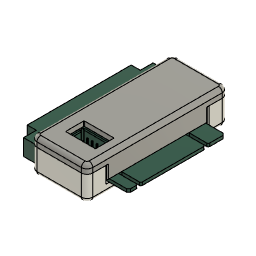
C64_Wifi_PET_adapter v4 (Autodesk Fusion 360 design; units mm, degrees)
Autodesk Fusion 360 part; units mm, degrees
sketch "pcb" plane through (0, 0, 0) normal (0, 0, 1) x (1, 0, 0) in component "PCB"
  arc A0 (28, 1.5) -> (27, 0.5) centre (28, 0.5) ccw
  line L0 (27, 0) -> (27, 0.5)
  line L1 (0, 54) -> (27, 54)
  line L2 (0, 54) -> (0, 0)
  line L3 (28, 1.5) -> (39, 1.5)
  line L4 (39.2, 42.04) -> (30, 42.04)
  line L5 (40, 51.5) -> (40, 44.44)
  line L6 (39, 1.5) -> (40, 2.5)
  line L7 (40, 4.12) -> (40, 5.6)
  arc A1 (30, 8) -> (29.2, 7.2) centre (30, 7.2) ccw
  arc A2 (29.2, 42.84) -> (30, 42.04) centre (30, 42.84) ccw
  arc A3 (30, 43.64) -> (29.2, 42.84) centre (30, 42.84) ccw
  line L8 (40, 4.12) -> (40, 2.5)
  arc A4 (40, 41.24) -> (39.2, 42.04) centre (39.2, 41.24) ccw
  arc A5 (29.2, 7.2) -> (30, 6.4) centre (30, 7.2) ccw
  line L9 (30, 8) -> (39.2, 8)
  line L10 (30, 43.64) -> (39.2, 43.64)
  line L11 (28, 52.5) -> (39, 52.5)
  arc A6 (39.2, 8) -> (40, 8.8) centre (39.2, 8.8) ccw
  arc A7 (27, 53.5) -> (28, 52.5) centre (28, 53.5) ccw
  arc A8 (39.2, 43.64) -> (40, 44.44) centre (39.2, 44.44) ccw
  line L12 (39, 52.5) -> (40, 51.5)
  line L13 (40, 8.8) -> (40, 41.24)
  line L14 (27, 54) -> (27, 53.5)
  line L15 (39.2, 6.4) -> (30, 6.4)
  arc A9 (40, 5.6) -> (39.2, 6.4) centre (39.2, 5.6) ccw
  line L16 (0, 0) -> (27, 0)
  line L17 (0.1, 41.86) -> (4, 41.86)
  line L18 (18.794, 6.016) -> (18.794, 6.524)
  line L19 (0.1, 35.9) -> (4, 35.9)
  line L20 (0.1, 43.82) -> (4, 43.82)
  line L21 (3, 49.28) -> (2, 49.28)
  arc A10 (4, 43.82) -> (4, 45.82) centre (4, 44.82) ccw
  arc A11 (4, 35.9) -> (4, 37.9) centre (4, 36.9) ccw
  line L22 (16.254, 3.476) -> (16.254, 3.984)
  line L23 (3, 41.36) -> (2, 41.36)
  line L24 (16.254, 3.984) -> (15.746, 3.984)
  line L25 (0.1, 45.82) -> (4, 45.82)
  line L26 (18.794, 3.476) -> (18.794, 3.984)
  arc A12 (3, 36.4) -> (3, 37.4) centre (3, 36.9) ccw
  line L27 (13.206, 6.016) -> (13.714, 6.016)
  line L28 (13.714, 3.476) -> (13.714, 3.984)
  arc A13 (3, 44.32) -> (3, 45.32) centre (3, 44.82) ccw
  arc A14 (2, 45.32) -> (2, 44.32) centre (2, 44.82) ccw
  line L29 (18.794, 3.984) -> (18.286, 3.984)
  line L30 (0.1, 37.9) -> (4, 37.9)
  line L31 (18.794, 6.524) -> (18.286, 6.524)
  line L32 (15.746, 6.524) -> (15.746, 6.016)
  line L33 (13.714, 6.524) -> (13.206, 6.524)
  line L34 (0.1, 49.78) -> (4, 49.78)
  line L35 (0.1, 39.86) -> (4, 39.86)
  line L36 (13.714, 3.984) -> (13.206, 3.984)
  line L37 (18.286, 6.524) -> (18.286, 6.016)
  line L38 (18.286, 3.984) -> (18.286, 3.476)
  line L39 (3, 37.4) -> (2, 37.4)
  line L40 (15.746, 6.016) -> (16.254, 6.016)
  line L41 (13.714, 6.016) -> (13.714, 6.524)
  line L42 (3, 48.28) -> (2, 48.28)
  arc A15 (2, 41.36) -> (2, 40.36) centre (2, 40.86) ccw
  arc A16 (4, 39.86) -> (4, 41.86) centre (4, 40.86) ccw
  arc A17 (3, 48.28) -> (3, 49.28) centre (3, 48.78) ccw
  arc A18 (3, 40.36) -> (3, 41.36) centre (3, 40.86) ccw
  line L43 (13.206, 6.524) -> (13.206, 6.016)
  arc A19 (2, 37.4) -> (2, 36.4) centre (2, 36.9) ccw
  line L44 (16.254, 6.524) -> (15.746, 6.524)
  line L45 (0.1, 47.78) -> (4, 47.78)
  arc A20 (2, 49.28) -> (2, 48.28) centre (2, 48.78) ccw
  line L46 (3, 44.32) -> (2, 44.32)
  line L47 (3, 36.4) -> (2, 36.4)
  line L48 (13.206, 3.476) -> (13.714, 3.476)
  line L49 (3, 40.36) -> (2, 40.36)
  line L50 (13.206, 3.984) -> (13.206, 3.476)
  arc A21 (4, 47.78) -> (4, 49.78) centre (4, 48.78) ccw
  line L51 (15.746, 3.476) -> (16.254, 3.476)
  line L52 (15.746, 3.984) -> (15.746, 3.476)
  line L53 (18.286, 6.016) -> (18.794, 6.016)
  line L54 (16.254, 6.016) -> (16.254, 6.524)
  line L55 (18.286, 3.476) -> (18.794, 3.476)
  line L56 (3, 45.32) -> (2, 45.32)
  line L57 (3, 32.44) -> (2, 32.44)
  arc A22 (2, 17.6) -> (2, 16.6) centre (2, 17.1) ccw
  line L58 (3, 29.48) -> (2, 29.48)
  arc A23 (3, 8.68) -> (3, 9.68) centre (3, 9.18) ccw
  line L59 (3, 25.52) -> (2, 25.52)
  line L60 (0.1, 14.14) -> (4, 14.14)
  line L61 (0.1, 24.02) -> (4, 24.02)
  arc A24 (2, 33.44) -> (2, 32.44) centre (2, 32.94) ccw
  line L62 (3, 12.64) -> (2, 12.64)
  line L63 (0.1, 6.22) -> (4, 6.22)
  arc A25 (4, 16.1) -> (4, 18.1) centre (4, 17.1) ccw
  line L64 (0.1, 20.06) -> (4, 20.06)
  arc A26 (2, 29.48) -> (2, 28.48) centre (2, 28.98) ccw
  line L65 (0.1, 29.98) -> (4, 29.98)
  arc A27 (3, 20.56) -> (3, 21.56) centre (3, 21.06) ccw
  line L66 (0.1, 10.18) -> (4, 10.18)
  arc A28 (4, 24.02) -> (4, 26.02) centre (4, 25.02) ccw
  arc A29 (3, 24.52) -> (3, 25.52) centre (3, 25.02) ccw
  arc A30 (4, 27.98) -> (4, 29.98) centre (4, 28.98) ccw
  line L67 (3, 9.68) -> (2, 9.68)
  arc A31 (2, 13.64) -> (2, 12.64) centre (2, 13.14) ccw
  line L68 (3, 20.56) -> (2, 20.56)
  line L69 (0.1, 33.94) -> (4, 33.94)
  line L70 (3, 5.72) -> (2, 5.72)
  line L71 (3, 16.6) -> (2, 16.6)
  arc A32 (3, 12.64) -> (3, 13.64) centre (3, 13.14) ccw
  arc A33 (2, 5.72) -> (2, 4.72) centre (2, 5.22) ccw
  line L72 (0.1, 16.1) -> (4, 16.1)
  arc A34 (2, 21.56) -> (2, 20.56) centre (2, 21.06) ccw
  line L73 (3, 8.68) -> (2, 8.68)
  arc A35 (4, 20.06) -> (4, 22.06) centre (4, 21.06) ccw
  line L74 (0.1, 12.14) -> (4, 12.14)
  line L75 (3, 4.72) -> (2, 4.72)
  line L76 (0.1, 8.18) -> (4, 8.18)
  arc A36 (2, 25.52) -> (2, 24.52) centre (2, 25.02) ccw
  arc A37 (4, 12.14) -> (4, 14.14) centre (4, 13.14) ccw
  arc A38 (2, 9.68) -> (2, 8.68) centre (2, 9.18) ccw
  line L77 (0.1, 31.94) -> (4, 31.94)
  arc A39 (4, 31.94) -> (4, 33.94) centre (4, 32.94) ccw
  arc A40 (4, 8.18) -> (4, 10.18) centre (4, 9.18) ccw
  arc A41 (4, 4.22) -> (4, 6.22) centre (4, 5.22) ccw
  line L78 (3, 21.56) -> (2, 21.56)
  line L79 (0.1, 18.1) -> (4, 18.1)
  arc A42 (3, 28.48) -> (3, 29.48) centre (3, 28.98) ccw
  arc A43 (3, 4.72) -> (3, 5.72) centre (3, 5.22) ccw
  arc A44 (3, 16.6) -> (3, 17.6) centre (3, 17.1) ccw
  line L80 (0.1, 4.22) -> (4, 4.22)
  line L81 (3, 13.64) -> (2, 13.64)
  line L82 (0.1, 27.98) -> (4, 27.98)
  line L83 (3, 24.52) -> (2, 24.52)
  line L84 (3, 28.48) -> (2, 28.48)
  arc A45 (3, 32.44) -> (3, 33.44) centre (3, 32.94) ccw
  line L85 (3, 17.6) -> (2, 17.6)
  line L86 (0.1, 26.02) -> (4, 26.02)
  line L87 (3, 33.44) -> (2, 33.44)
  line L88 (0.1, 22.06) -> (4, 22.06)
  line L89 (14.73, 1.6662) -> (14.73, 1.19)
  line L90 (23.62, 6.7463) -> (23.62, 0.3962)
  arc A46 (22.35, 9.6038) -> (21.08, 9.6038) centre (21.715, 9.6038) ccw
  line L91 (14.73, 1.6662) -> (9.65, 1.6662)
  line L92 (9.1737, 6.7463) -> (9.1737, 1.19)
  line L93 (8.38, 8.175) -> (8.38, 9.6038)
  line L94 (14.73, 1.19) -> (14.73, 0.3962)
  line L95 (22.35, 1.6662) -> (22.8263, 1.19)
  line L96 (22.35, 8.175) -> (22.35, 6.7463)
  line L97 (9.65, 8.175) -> (9.1737, 8.175)
  line L98 (22.8263, 8.175) -> (22.8263, 8.81)
  line L99 (9.1737, 1.19) -> (9.65, 1.6662)
  line L100 (9.1737, 8.81) -> (9.65, 8.3338)
  line L101 (22.35, 8.175) -> (22.8263, 8.175)
  line L102 (8.38, 0.3962) -> (8.38, 6.7463)
  line L103 (14.73, 1.19) -> (9.1737, 1.19)
  line L104 (23.62, 9.6038) -> (23.62, 8.175)
  arc A47 (10.92, 9.6038) -> (9.65, 9.6038) centre (10.285, 9.6038) ccw
  line L105 (22.8263, 8.175) -> (23.62, 8.175)
  line L106 (22.35, 6.7463) -> (22.8263, 6.7463)
  line L107 (9.65, 1.6662) -> (9.65, 6.7463)
  line L108 (9.1737, 8.81) -> (9.1737, 8.175)
  arc A48 (16.4763, 9.6038) -> (15.3651, 9.6038) centre (15.9207, 9.6038) ccw
  line L109 (22.35, 1.6662) -> (17.27, 1.6662)
  line L110 (9.65, 8.3338) -> (22.35, 8.3338)
  line L111 (22.8263, 6.7463) -> (22.8263, 1.19)
  line L112 (17.27, 1.19) -> (22.8263, 1.19)
  line L113 (22.35, 6.7463) -> (22.35, 1.6662)
  line L114 (9.1737, 8.175) -> (8.38, 8.175)
  line L115 (0.1, 20.06) -> (-1, 20.06)
  line L116 (0.1, 49.78) -> (-1, 49.78)
  line L117 (-1, 53.8) -> (0, 53.8)
  line L118 (0, 27.25) -> (-1, 27.25)
  line L119 (-1, 14.87) -> (0, 14.87)
  line L120 (0.1, 35.9) -> (-1, 35.9)
  line L121 (0, 50.51) -> (0, 51.01)
  line L122 (0, 42.59) -> (0, 43.09)
  line L123 (0.1, 41.86) -> (-1, 41.86)
  line L124 (0.1, 47.78) -> (-1, 47.78)
  line L125 (0, 61.25) -> (-6.8, 61.25)
  line L126 (-1, 18.83) -> (0, 18.83)
  line L127 (0.1, 43.82) -> (-1, 43.82)
  line L128 (0, 31.21) -> (-1, 31.21)
  line L129 (0, -7.25) -> (-6.8, -7.25)
  line L130 (0, 23.29) -> (-1, 23.29)
  line L131 (0.1, 14.14) -> (-1, 14.14)
  line L132 (0.1, 29.98) -> (-1, 29.98)
  line L133 (-1, 42.59) -> (0, 42.59)
  line L134 (0, 59.7) -> (0, 61.25)
  line L135 (0, 0.2) -> (-1, 0.2)
  line L136 (0.1, 22.06) -> (-1, 22.06)
  line L137 (0.1, 39.86) -> (-1, 39.86)
  line L138 (0, 15.37) -> (-1, 15.37)
  line L139 (0, 58) -> (-2.8667, 58)
  line L140 (-1.6, -2.3) -> (0, -2.3)
  line L141 (0, 51.01) -> (-1, 51.01)
  line L142 (-6.8, 56.3) -> (-6.8, 59.7)
  line L143 (0, -2.3) -> (0, 0.2)
  line L144 (0.1, 45.82) -> (-1, 45.82)
  line L145 (0, 56.3) -> (0, 58)
  line L146 (0, -5.7) -> (0, -4)
  line L147 (-11.6, 54.5) -> (-6.8, 54.5)
  line L148 (0, 19.33) -> (-1, 19.33)
  line L149 (-1, 30.71) -> (0, 30.71)
  line L150 (-1, 50.51) -> (0, 50.51)
  line L151 (0, 43.09) -> (-1, 43.09)
  line L152 (0, -7.25) -> (0, -5.7)
  line L153 (0, 46.55) -> (0, 47.05)
  line L154 (-1, 0.2) -> (-1, 53.8)
  line L155 (-1, 38.63) -> (0, 38.63)
  line L156 (0, 39.13) -> (-1, 39.13)
  line L157 (0.1, 37.9) -> (-1, 37.9)
  line L158 (-1, 46.55) -> (0, 46.55)
  line L159 (0, 53.8) -> (0, 56.3)
  line L160 (-11.6, -4) -> (-8.7333, -4)
  line L161 (0.1, 18.1) -> (-1, 18.1)
  line L162 (0.1, 24.02) -> (-1, 24.02)
  line L163 (-11.6, -0.5) -> (-11.6, 54.5)
  line L164 (0, 38.63) -> (0, 39.13)
  line L165 (0, 58) -> (0, 59.7)
  line L166 (0, 47.05) -> (-1, 47.05)
  line L167 (-3.548, 58) -> (-3.6853, 58)
  line L168 (-6.8, 54.5) -> (-6.8, 56.3)
  line L169 (0.1, 26.02) -> (-1, 26.02)
  line L170 (0, -4) -> (0, -2.3)
  line L171 (-1, 22.79) -> (0, 22.79)
  line L172 (0.1, 27.98) -> (-1, 27.98)
  line L173 (0, 26.75) -> (0, 27.25)
  line L174 (-8.7333, 58) -> (-11.6, 58)
  line L175 (-6.8, -2.3) -> (-5.2, -2.3)
  line L176 (-4.2, -5.7) -> (-2.6, -5.7)
  line L177 (-3.6853, -4) -> (-3.548, -4)
  line L178 (-6.8, 56.3) -> (-5.2, 56.3)
  line L179 (22.35, 8.3338) -> (22.35, 8.175)
  line L180 (9.65, 8.175) -> (9.65, 8.3338)
  line L181 (22.35, 8.3338) -> (22.8263, 8.81)
  line L182 (-6.8, -7.25) -> (-6.8, -5.7)
  line L183 (17.27, 1.19) -> (17.27, 0.3962)
  line L184 (9.1737, 8.81) -> (22.8263, 8.81)
  line L185 (8.38, 6.7463) -> (8.38, 8.175)
  line L186 (-4.2, 56.3) -> (-2.6, 56.3)
  line L187 (9.65, 6.7463) -> (9.1737, 6.7463)
  line L188 (-6.8, -0.5) -> (-11.6, -0.5)
  line L189 (-6.8, -2.3) -> (-6.8, -0.5)
  line L190 (23.62, 0.3962) -> (17.27, 0.3962)
  line L191 (9.1737, 6.7463) -> (8.38, 6.7463)
  line L192 (-1.6, 59.7) -> (0, 59.7)
  line L193 (-4.2, 59.7) -> (-2.6, 59.7)
  line L194 (17.27, 1.6662) -> (14.73, 1.6662)
  line L195 (-8.052, -4) -> (-7.9147, -4)
  line L196 (8.38, 9.6038) -> (23.62, 9.6038)
  line L197 (14.73, 0.3962) -> (8.38, 0.3962)
  line L198 (-2.8667, -4) -> (0, -4)
  line L199 (-6.8, 59.7) -> (-5.2, 59.7)
  line L200 (-6.8, -5.7) -> (-5.2, -5.7)
  line L201 (9.65, 6.7463) -> (9.65, 8.175)
  line L202 (-4.2, -2.3) -> (-2.6, -2.3)
  line L203 (22.8263, 6.7463) -> (23.62, 6.7463)
  line L204 (17.27, 1.6662) -> (17.27, 1.19)
  line L205 (23.62, 8.175) -> (23.62, 6.7463)
  line L206 (17.27, 0.3962) -> (14.73, 0.3962)
  line L207 (-1.6, -5.7) -> (0, -5.7)
  line L208 (-6.8, 59.7) -> (-6.8, 61.25)
  line L209 (-7.2333, -4) -> (-4.3667, -4)
  line L210 (-7.9147, 58) -> (-8.052, 58)
  line L211 (-4.3667, 58) -> (-7.2333, 58)
  line L212 (-1.6, 56.3) -> (0, 56.3)
  line L213 (-6.8, -5.7) -> (-6.8, -2.3)
  line L214 (0.1, 8.18) -> (-1, 8.18)
  line L215 (0, 11.41) -> (-1, 11.41)
  line L216 (0.1, 12.14) -> (-1, 12.14)
  line L217 (0, 6.95) -> (0, 7.45)
  line L218 (0.1, 10.18) -> (-1, 10.18)
  line L219 (0.1, 4.22) -> (-1, 4.22)
  line L220 (0, 7.45) -> (-1, 7.45)
  line L221 (0.1, 6.22) -> (-1, 6.22)
  line L222 (-1, 2.99) -> (0, 2.99)
  line L223 (0, 2.99) -> (0, 3.49)
  line L224 (0.1, 16.1) -> (-1, 16.1)
  line L225 (-1, 10.91) -> (0, 10.91)
  line L226 (-1, 26.75) -> (0, 26.75)
  line L227 (-1, 34.67) -> (0, 34.67)
  line L228 (-1, 6.95) -> (0, 6.95)
  line L229 (0, 34.67) -> (0, 35.17)
  line L230 (0, 35.17) -> (-1, 35.17)
  line L231 (0, 3.49) -> (-1, 3.49)
  line L232 (0, 18.83) -> (0, 19.33)
  line L233 (0.1, 31.94) -> (-1, 31.94)
  line L234 (0, 22.79) -> (0, 23.29)
  line L235 (0.1, 33.94) -> (-1, 33.94)
  line L236 (0, 30.71) -> (0, 31.21)
  line L237 (0, 14.87) -> (0, 15.37)
  line L238 (0, 10.91) -> (0, 11.41)
  arc A49 (3, 48.28) -> (3, 49.28) centre (3, 48.78) ccw
  line L239 (3, 37.4) -> (2, 37.4)
  arc A50 (2, 41.36) -> (2, 40.36) centre (2, 40.86) ccw
  line L240 (0.1, 33.94) -> (4, 33.94)
  line L241 (3, 32.44) -> (2, 32.44)
  arc A51 (4, 39.86) -> (4, 41.86) centre (4, 40.86) ccw
  arc A52 (3, 32.44) -> (3, 33.44) centre (3, 32.94) ccw
  arc A53 (4, 31.94) -> (4, 33.94) centre (4, 32.94) ccw
  line L242 (3, 33.44) -> (2, 33.44)
  arc A54 (2, 45.32) -> (2, 44.32) centre (2, 44.82) ccw
  line L243 (0.1, 31.94) -> (4, 31.94)
  arc A55 (2, 49.28) -> (2, 48.28) centre (2, 48.78) ccw
  line L244 (0.1, 29.98) -> (4, 29.98)
  line L245 (0.1, 35.9) -> (4, 35.9)
  line L246 (3, 41.36) -> (2, 41.36)
  arc A56 (4, 35.9) -> (4, 37.9) centre (4, 36.9) ccw
  line L247 (0.1, 41.86) -> (4, 41.86)
  arc A57 (4, 43.82) -> (4, 45.82) centre (4, 44.82) ccw
  line L248 (0.1, 37.9) -> (4, 37.9)
  arc A58 (3, 44.32) -> (3, 45.32) centre (3, 44.82) ccw
  line L249 (0.1, 4.22) -> (4, 4.22)
  arc A59 (2, 21.56) -> (2, 20.56) centre (2, 21.06) ccw
  arc A60 (3, 24.52) -> (3, 25.52) centre (3, 25.02) ccw
  arc A61 (2, 33.44) -> (2, 32.44) centre (2, 32.94) ccw
  line L250 (3, 49.28) -> (2, 49.28)
  line L251 (3, 36.4) -> (2, 36.4)
  line L252 (3, 40.36) -> (2, 40.36)
  arc A62 (2, 37.4) -> (2, 36.4) centre (2, 36.9) ccw
  line L253 (0.1, 43.82) -> (4, 43.82)
  line L254 (0.1, 49.78) -> (4, 49.78)
  line L255 (3, 45.32) -> (2, 45.32)
  line L256 (0.1, 45.82) -> (4, 45.82)
  arc A63 (4, 47.78) -> (4, 49.78) centre (4, 48.78) ccw
  line L257 (0.1, 47.78) -> (4, 47.78)
  arc A64 (3, 28.48) -> (3, 29.48) centre (3, 28.98) ccw
  arc A65 (3, 40.36) -> (3, 41.36) centre (3, 40.86) ccw
  line L258 (0.1, 22.06) -> (4, 22.06)
  line L259 (0.1, 10.18) -> (4, 10.18)
  line L260 (3, 44.32) -> (2, 44.32)
  line L261 (0.1, 8.18) -> (4, 8.18)
  arc A66 (2, 13.64) -> (2, 12.64) centre (2, 13.14) ccw
  line L262 (3, 17.6) -> (2, 17.6)
  line L263 (3, 12.64) -> (2, 12.64)
  arc A67 (3, 36.4) -> (3, 37.4) centre (3, 36.9) ccw
  arc A68 (4, 8.18) -> (4, 10.18) centre (4, 9.18) ccw
  line L264 (3, 48.28) -> (2, 48.28)
  line L265 (0.1, 39.86) -> (4, 39.86)
  arc A69 (2, 29.48) -> (2, 28.48) centre (2, 28.98) ccw
  arc A70 (2, 9.68) -> (2, 8.68) centre (2, 9.18) ccw
  arc A71 (3, 4.72) -> (3, 5.72) centre (3, 5.22) ccw
  line L266 (0.1, 14.14) -> (4, 14.14)
  line L267 (3, 9.68) -> (2, 9.68)
  line L268 (0.1, 27.98) -> (4, 27.98)
  line L269 (3, 21.56) -> (2, 21.56)
  line L270 (0.1, 24.02) -> (4, 24.02)
  arc A72 (4, 16.1) -> (4, 18.1) centre (4, 17.1) ccw
  line L271 (0.1, 16.1) -> (4, 16.1)
  line L272 (0.1, 12.14) -> (4, 12.14)
  arc A73 (3, 12.64) -> (3, 13.64) centre (3, 13.14) ccw
  line L273 (3, 13.64) -> (2, 13.64)
  line L274 (3, 29.48) -> (2, 29.48)
  arc A74 (3, 8.68) -> (3, 9.68) centre (3, 9.18) ccw
  line L275 (3, 16.6) -> (2, 16.6)
  line L276 (0.1, 26.02) -> (4, 26.02)
  arc A75 (4, 20.06) -> (4, 22.06) centre (4, 21.06) ccw
  arc A76 (3, 16.6) -> (3, 17.6) centre (3, 17.1) ccw
  line L277 (3, 8.68) -> (2, 8.68)
  arc A77 (2, 25.52) -> (2, 24.52) centre (2, 25.02) ccw
  line L278 (3, 5.72) -> (2, 5.72)
  line L279 (0.1, 18.1) -> (4, 18.1)
  arc A78 (3, 20.56) -> (3, 21.56) centre (3, 21.06) ccw
  line L280 (3, 25.52) -> (2, 25.52)
  arc A79 (4, 27.98) -> (4, 29.98) centre (4, 28.98) ccw
  line L281 (0.1, 20.06) -> (4, 20.06)
  arc A80 (2, 17.6) -> (2, 16.6) centre (2, 17.1) ccw
  line L282 (0.1, 6.22) -> (4, 6.22)
  arc A81 (2, 5.72) -> (2, 4.72) centre (2, 5.22) ccw
  arc A82 (4, 12.14) -> (4, 14.14) centre (4, 13.14) ccw
  line L283 (3, 28.48) -> (2, 28.48)
  line L284 (3, 20.56) -> (2, 20.56)
  line L285 (3, 4.72) -> (2, 4.72)
  line L286 (3, 24.52) -> (2, 24.52)
  arc A83 (4, 4.22) -> (4, 6.22) centre (4, 5.22) ccw
  arc A84 (4, 24.02) -> (4, 26.02) centre (4, 25.02) ccw
  point P0 (16, 5)
  point P1 (0.4763, 51.9113)
  point P2 (0, 27)
  point P3 (40, 27)
extrude "Extrude1" add sketch "pcb" against normal blind 1.6 contours A0 L0 L1 L2 L3 L4 L5 L6 L7 A1 A2 A3 L8 A4 A5 L9 L10 L11 A6 A7 A8 L12 L13 L14 L15 A9 L16 L17 L19 L20 A10 A11 L25 L30 L34 L35 A16 L45 A21 L60 L61 L63 A25 L64 L65 L66 A28 A30 L69 L72 A35 L74 L76 A37 L77 A39 A40 A41 L79 L80 L82 L86 L88 L115 L116 L120 L121 L122 L123 L124 L127 L131 L132 L136 L137 L143 L144 L153 L157 L159 L161 L162 L164 L169 L172 L173 L214 L216 L217 L218 L219 L221 L223 L224 L229 L232 L233 L234 L235 L236 L237 L238 L240 A51 A53 L243 L244 L245 A56 L247 A57 L248 L249 L253 L254 L256 A63 L257 L258 L259 L261 A68 L265 L266 L268 L270 A72 L271 L272 L276 A75 L279 A79 L281 L282 A82 A83 A84 | L2 L63 A41 L80 L219 L221 L249 L282 A83 | L2 L66 L76 A40 L214 L218 L259 L261 A68 | L2 L60 L74 A37 L131 L216 L266 L272 A82 | L2 A25 L72 L79 L161 L224 A72 L271 L279 | L2 L64 A35 L88 L115 L136 L258 A75 L281 | L2 L61 A28 L86 L162 L169 L270 L276 A84 | L2 L34 L45 A21 L116 L124 L254 A63 L257 | L2 L65 A30 L82 L132 L172 L244 L268 A79 | L2 L20 A10 L25 L127 L144 A57 L253 L256 | L2 L69 L77 A39 L233 L235 L240 A53 L243 | L2 L17 L35 A16 L123 L137 A51 L247 L265 | L2 L19 A11 L30 L120 L157 L245 A56 L248 | L18 L31 L37 L53 | L21 L42 A17 A20 A49 A55 L250 L264 | L22 L24 L51 L52 | L23 A15 A18 L49 A50 L246 L252 A65 | L26 L29 L38 L55 | A12 L39 A19 L47 L239 L251 A62 A67 | L27 L33 L41 L43 | L28 L36 L48 L50 | A13 A14 L46 L56 A54 A58 L255 L260 | L32 L40 L44 L54 | L57 A24 A45 L87 L241 A52 L242 A61 | A22 L71 A44 L85 L262 L275 A76 A80 | L58 A26 A42 L84 A64 A69 L274 L283 | A23 L67 L73 A38 A70 L267 A74 L277 | L59 A29 A36 L83 A60 A77 L280 L286 | L62 A31 A32 L81 A66 L263 A73 L273 | A27 L68 A34 L78 A59 L269 A78 L284 | L70 A33 L75 A43 A71 L278 A81 L285 | L89 L94 L183 L194 L204 L206 | L89 L91 L99 L103 | L91 L96 L107 L109 L110 L113 L179 L180 L194 L201 | L92 L94 L102 L103 L191 L197 | L92 L99 L107 L187 | L95 L109 L112 L204 | L97 L114 L185 L187 L191 L201 | L95 L106 L111 L113 | L90 L111 L112 L183 L190 L203 | L97 L100 L108 L180 | L96 L101 L105 L106 L203 L205 | L93 L98 L104 L105 L108 L114 L184 L196 | L100 L110 L181 L184 | L98 L101 L179 L181 | A47 L196 | A46 L196 | A48 L196 makes body 1 in component "PCB"
extrude "Extrude2" add sketch "pcb" along normal blind 0.5 contours L2 L154 L219 L221 | L2 L63 A41 L80 L219 L221 L249 L282 A83 | L2 L154 L214 L218 | L2 L66 L76 A40 L214 L218 L259 L261 A68 | L2 L131 L154 L216 | L2 L60 L74 A37 L131 L216 L266 L272 A82 | L2 L154 L161 L224 | L2 A25 L72 L79 L161 L224 A72 L271 L279 | L2 L115 L136 L154 | L2 L64 A35 L88 L115 L136 L258 A75 L281 | L2 L154 L162 L169 | L2 L61 A28 L86 L162 L169 L270 L276 A84 | L2 L34 L45 A21 L116 L124 L254 A63 L257 | L2 L116 L124 L154 | L2 L132 L154 L172 | L2 L65 A30 L82 L132 L172 L244 L268 A79 | L2 L20 A10 L25 L127 L144 A57 L253 L256 | L2 L127 L144 L154 | L2 L154 L233 L235 | L2 L69 L77 A39 L233 L235 L240 A53 L243 | L2 L17 L35 A16 L123 L137 A51 L247 L265 | L2 L123 L137 L154 | L2 L120 L154 L157 | L2 L19 A11 L30 L120 L157 L245 A56 L248 bodies 1 in component "PCB"
extrude "Extrude3" add sketch "pcb" along normal blind 4.9 and the other way blind 3.7 contours L2 L117 L125 L129 L134 L135 L142 L143 L145 L146 L147 L152 L154 L159 L163 L165 L168 L170 L182 L188 L189 L208 L213 | L2 L154 L222 L223 L231 | L2 L154 L217 L220 L228 | L2 L154 L215 L225 L238 | L2 L119 L138 L154 L237 | L2 L126 L148 L154 L232 | L2 L130 L154 L171 L234 | L2 L121 L141 L150 L154 | L2 L118 L154 L173 L226 | L2 L153 L154 L158 L166 | L2 L128 L149 L154 L236 | L2 L122 L133 L151 L154 | L2 L154 L227 L229 L230 | L2 L154 L155 L156 L164 bodies 1 in component "PCB"
extrude "Extrude4" add sketch "pcb" along normal blind 9.2 contours L89 L91 L99 L103 | L92 L94 L102 L103 L191 L197 | L92 L99 L107 L187 | L95 L109 L112 L204 | L95 L106 L111 L113 | L90 L111 L112 L183 L190 L203 | L97 L100 L108 L180 | L93 L98 L104 L105 L108 L114 L184 L196 | L100 L110 L181 L184 | L98 L101 L179 L181 bodies 1 in component "PCB"
chamfer "Chamfer1" distance 0.476 angle 45 7 edges at (9.65, 4.2063, 9.2) (12.19, 1.6662, 9.2) (19.81, 1.6662, 9.2) (22.35, 4.2063, 9.2) (22.35, 8.2544, 9.2) (16, 8.3338, 9.2) (9.65, 8.2544, 9.2) on bodies 1 in component "PCB"
extrude "Extrude5" add sketch "pcb" along normal blind 2.3 contours L89 L94 L183 L194 L204 L206 | L91 L96 L107 L109 L110 L113 L179 L180 L194 L201 | L97 L114 L185 L187 L191 L201 | L96 L101 L105 L106 L203 L205 bodies 1 in component "PCB"
extrude "Extrude6" add sketch "pcb" along normal blind 8 contours L18 L31 L37 L53 | L22 L24 L51 L52 | L26 L29 L38 L55 | L27 L33 L41 L43 | L28 L36 L48 L50 | L32 L40 L44 L54 bodies 1 in component "PCB"
extrude "Extrude7" add sketch "pcb" along normal blind 8.2 contours A47 L196 | A46 L196 | A48 L196 bodies 1 in component "PCB"
fillet "Fillet1" radius 0.5 3 edges at (21.715, 10.2388, 8.2) (15.9207, 10.1594, 8.2) (10.285, 10.2388, 8.2) on bodies 1 in component "PCB"
sketch "connector_dril" plane through (-6.8, 0, 0) normal (-1, 0, 0) x (0, -1, 0) in component "PCB"
  line L0 (7.25, -3.7) -> (7.25, 4.9)
  line L1 (7.25, 4.9) -> (0.5, 4.9)
  line L2 (0.5, 4.9) -> (0.5, -3.7)
  line L3 (0.5, -3.7) -> (7.25, -3.7)
  line L4 (-61.25, 4.9) -> (-54.5, 4.9)
  line L5 (-61.25, -3.7) -> (-61.25, 4.9)
  line L6 (-54.5, -3.7) -> (-61.25, -3.7)
  line L7 (0.5, 4.9) -> (7.25, 4.9)
  line L8 (7.25, -3.7) -> (7.25, 4.9)
  line L9 (7.25, -3.7) -> (0.5, -3.7)
  line L10 (0.5, -3.7) -> (-54.5, -3.7)
  line L11 (-54.5, 4.9) -> (0.5, 4.9)
  line L12 (0.5, -3.7) -> (0.5, 4.9)
  line L13 (-54.5, -3.7) -> (-54.5, 4.9)
  line L14 (4, 4.9) -> (4, -3.7) construction
  line L15 (7.25, 0.6) -> (0.5, 0.6) construction
  circle A0 centre (4, 0.6) radius 1.65
  line L16 (-27, 4.9) -> (-27, -3.7) construction
  circle A1 centre (-58, 0.6) radius 1.65
  point P0 (4, 0)
  dimension "d21" = 3.3
  constraint coincident L7 L14.start
  constraint coincident L9 L14.end
  constraint perpendicular L9 L14
  constraint coincident P0 L14
  constraint midpoint L8 L15.start
  constraint midpoint L12 L15.end
  constraint midpoint L14 A0.centre
  constraint midpoint L11 L16.start
  constraint midpoint L10 L16.end
  constraint symmetric A0 L16 A1
  measures "d21" diameter of A0
extrude "Extrude8" cut sketch "connector_dril" against normal blind 6.8 contours A0 | A1 bodies 1 in component "PCB"
ref_plane "WorkPlane1" through (0, 0, -3.6) normal (0, 0, 1) x (1, 0, 0) in component "bottom shell"
sketch "bottom_shell" plane through (0, 0, -3.6) normal (0, 0, 1) x (1, 0, 0) in component "bottom shell"
  line L0 (0, -7.25) -> (-6.8, -7.25) construction
  line L1 (0, -7.25) -> (0, -5.7) construction
  line L2 (0, -5.7) -> (0, -4) construction
  line L3 (0, -4) -> (0, -2.3) construction
  line L4 (0, -2.3) -> (0, 0.2) construction
  line L5 (0, 0) -> (27, 0) construction
  line L6 (27, 0) -> (27, 0.5) construction
  line L7 (0, 54) -> (27, 54) construction
  line L8 (0, 53.8) -> (0, 56.3) construction
  line L9 (0, 56.3) -> (0, 58) construction
  line L10 (0, 58) -> (0, 59.7) construction
  line L11 (0, 59.7) -> (0, 61.25) construction
  line L12 (0, 61.25) -> (-6.8, 61.25) construction
  line L13 (27, 54) -> (27, 53.5) construction
  line L14 (0, -7.25) -> (0, 61.25) construction
  line L15 (0.3, 61.25) -> (0.3, -7.25)
  line L16 (0, 27) -> (31, 27) construction
  line L17 (27, 0) -> (27, 54) construction
  line L18 (3.3, 64.25) -> (26.8, 64.25)
  line L19 (29.8, 61.25) -> (29.8, -7.25)
  line L20 (26.8, -10.25) -> (3.3, -10.25)
  arc A0 (29.8, 61.25) -> (26.8, 64.25) centre (26.8, 61.25) ccw
  arc A1 (3.3, 64.25) -> (0.3, 61.25) centre (3.3, 61.25) ccw
  arc A2 (26.8, -10.25) -> (29.8, -7.25) centre (26.8, -7.25) ccw
  arc A3 (0.3, -7.25) -> (3.3, -10.25) centre (3.3, -7.25) ccw
  arc A4 (26.8, -7.75) -> (27.3, -7.25) centre (26.8, -7.25) ccw
  line L21 (27.3, 61.25) -> (27.3, -7.25)
  arc A5 (27.3, 61.25) -> (26.8, 61.75) centre (26.8, 61.25) ccw
  line L22 (3.3, 61.75) -> (26.8, 61.75)
  arc A6 (3.3, 61.75) -> (2.8, 61.25) centre (3.3, 61.25) ccw
  line L23 (2.8, 61.25) -> (2.8, -7.25)
  arc A7 (2.8, -7.25) -> (3.3, -7.75) centre (3.3, -7.25) ccw
  line L24 (26.8, -7.75) -> (3.3, -7.75)
  arc A8 (26.8, -8.75) -> (28.3, -7.25) centre (26.8, -7.25) ccw
  line L25 (28.3, 61.25) -> (28.3, -7.25)
  arc A9 (28.3, 61.25) -> (26.8, 62.75) centre (26.8, 61.25) ccw
  line L26 (3.3, 62.75) -> (26.8, 62.75)
  arc A10 (3.3, 62.75) -> (1.8, 61.25) centre (3.3, 61.25) ccw
  line L27 (1.8, 61.25) -> (1.8, -7.25)
  arc A11 (1.8, -7.25) -> (3.3, -8.75) centre (3.3, -7.25) ccw
  line L28 (26.8, -8.75) -> (3.3, -8.75)
  line L29 (2.8, 54.3) -> (0.3, 54.3)
  line L30 (27, 54) -> (29.8, 54) construction
  line L31 (27.3, 53.8) -> (29.8, 53.8)
  line L32 (27.3, 0.2) -> (29.8, 0.2)
  line L33 (2.8, -0.3) -> (0.3, -0.3)
  line L34 (10.3, 61.75) -> (7.8, 61.75)
  line L35 (7.8, 61.75) -> (7.8, 54.3)
  line L36 (7.8, 54.3) -> (10.3, 54.3)
  line L37 (10.3, 54.3) -> (10.3, 61.75)
  line L38 (10.3, -0.3) -> (10.3, -7.75)
  line L39 (7.8, -0.3) -> (10.3, -0.3)
  line L40 (7.8, -7.75) -> (7.8, -0.3)
  line L41 (27, 53.5) -> (29.8, 53.5) construction
  line L42 (10.3, 54.3) -> (7.8, 54.3)
  line L43 (7.8, 54.3) -> (7.8, 51.8)
  line L44 (7.8, 51.8) -> (10.3, 51.8)
  line L45 (10.3, 51.8) -> (10.3, 54.3)
  line L46 (10.3, 2.2) -> (10.3, -0.3)
  line L47 (7.8, 2.2) -> (10.3, 2.2)
  line L48 (7.8, -0.3) -> (7.8, 2.2)
  line L49 (10.3, 58.025) -> (26.7375, 58.025) construction
  circle A12 centre (21.3, 58.025) radius 3
  circle A13 centre (21.3, 58.025) radius 1.75
  line L50 (25, 58.025) -> (25, 61.75)
  line L51 (17.6, 58.025) -> (17.6, 61.75)
  line L52 (21.3, 58.025) -> (21.3, 61.75) construction
  arc A14 (17.6, 58.025) -> (25, 58.025) centre (21.3, 58.025) ccw construction
  arc A15 (17.6, 58.025) -> (25, 58.025) centre (21.3, 58.025) ccw
  line L53 (25, -4.025) -> (25, -7.75)
  line L54 (17.6, -4.025) -> (17.6, -7.75)
  arc A16 (25, -4.025) -> (17.6, -4.025) centre (21.3, -4.025) ccw
  circle A17 centre (21.3, -4.025) radius 3
  circle A18 centre (21.3, -4.025) radius 1.75
  line L55 (2.8, 54.3) -> (4.3, 54.3)
  line L56 (4.3, 54.3) -> (4.3, 61.75)
  line L57 (4.3, -0.3) -> (4.3, -7.75)
  line L58 (2.8, -0.3) -> (4.3, -0.3)
  dimension "d28" = 0.3
  dimension "d29" = 2.8
  dimension "d31" = 3
  dimension "d32" = 3
  dimension "d33" = 2.5
  dimension "d34" = 1.5
  dimension "d35" = 0.3
  dimension "d37" = 2.5
  dimension "d38" = 0.3
  dimension "d41" = 0.3
  dimension "d42" = 5
  dimension "d43" = 2.5
  dimension "d44" = 6
  dimension "d45" = 6
  dimension "d46" = 3.5
  dimension "d49" = 0.7
  dimension "d65" = 1.5
  constraint coincident L0.start L1.start
  constraint coincident L11.end L12.start
  constraint perpendicular L12 L15
  constraint midpoint L14 L16.start
  constraint perpendicular L15 L16
  constraint coincident L5.end L6.start
  constraint coincident L7.end L13.start
  constraint perpendicular L15 L18
  constraint perpendicular L18 L19
  constraint perpendicular L15 L20
  constraint tangent L19 A0
  constraint tangent L18 A0
  constraint tangent L15 A1
  constraint tangent L18 A1
  constraint equal A0 A1
  constraint tangent L19 A2
  constraint tangent L20 A2
  constraint equal A0 A2
  constraint tangent L15 A3
  constraint tangent L20 A3
  constraint equal A0 A3
  constraint symmetric L16 L18 L20
  constraint coincident L23 L29.start
  constraint coincident L15 L29.end
  constraint perpendicular L15 L29
  constraint coincident L19 L30.end
  constraint perpendicular L19 L30
  constraint coincident L21 L31.start
  constraint coincident L19 L31.end
  constraint perpendicular L19 L31
  constraint symmetric L16 L29.start L33.start
  constraint symmetric L16 L29.end L33.end
  constraint symmetric L16 L31.start L32.start
  constraint symmetric L16 L31.end L32.end
  constraint horizontal L34
  constraint vertical L35
  constraint horizontal L36
  constraint vertical L37
  constraint coincident L22 L34.start
  constraint symmetric L16 L34.start L38.end
  constraint symmetric L16 L34.end L40.start
  constraint symmetric L16 L35.end L39.start
  constraint symmetric L16 L36.end L38.start
  constraint coincident L13.end L41.start
  constraint coincident L19 L41.end
  constraint perpendicular L19 L41
  constraint horizontal L42
  constraint vertical L43
  constraint horizontal L44
  constraint vertical L45
  constraint collinear L35 L43
  constraint symmetric L16 L43.end L47.start
  constraint symmetric L16 L44.end L46.start
  constraint midpoint L37 L49.start
  constraint perpendicular L21 L49
  constraint coincident L49 A12.centre
  constraint concentric A12 A13
  constraint coincident L49 L50.start
  constraint coincident L22 L50.end
  constraint perpendicular L22 L50
  constraint coincident L49 L51.start
  constraint coincident L22 L51.end
  constraint perpendicular L22 L51
  constraint coincident A12.centre A13.centre
  constraint coincident L22 L52.end
  constraint perpendicular L22 L52
  constraint tangent L51 A14
  constraint concentric A12 A15
  constraint coincident L50 A14.end
  constraint coincident L51 A14.start
  constraint tangent L51 A15
  constraint tangent L50 A15
  constraint symmetric L16 A12 A17
  constraint symmetric L16 A13 A18
  constraint symmetric L16 L50.start L53.start
  constraint symmetric L16 L50.end L53.end
  constraint symmetric L16 L51.start L54.start
  constraint symmetric L16 L51.end L54.end
  constraint symmetric L16 A15 A16
  constraint perpendicular L23 L55
  constraint coincident L22 L56.end
  constraint perpendicular L22 L56
  constraint symmetric L16 L55.end L57.start
  constraint symmetric L16 L56.end L57.end
  measures "d28" distance of L14 L15
  measures "d29" distance of L17 L19
  measures "d31" radius of A0
  measures "d32" distance of L12 L18
  measures "d35" distance of L7 L29
  measures "d37" distance of L35 L37
  measures "d38" distance of L7 L36
  measures "d41" distance of L31 L41
  measures "d42" distance of L23 L35
  measures "d43" distance of L42 L44
  measures "d44" diameter of A12
  measures "d45" distance of L21 A12.centre
  measures "d46" diameter of A13
  measures "d49" distance of A12 A15
  measures "d65" distance of L23 L56
extrude "Extrude1'" add sketch "bottom_shell" against normal blind 2.5 separate body contours L15 L18 L19 A0 A1 L25 A9 L26 A10 L27 L29 L31 | L15 L27 L29 L33 | L15 L19 L20 A2 A3 A8 L25 L27 A11 L28 L32 L33 | L23 L27 L29 L33 | L21 A5 L22 A6 L23 L25 A9 L26 A10 L27 L29 L31 L34 | A4 L21 L23 A7 L24 A8 L25 L27 A11 L28 L32 L33 | A4 L21 A5 L22 L23 L24 L35 L37 L38 L40 L43 L44 L45 L46 L47 L48 L50 L51 A15 L53 L54 A16 L55 L56 L57 L58 | L22 A6 L23 L55 L56 | L23 A7 L24 L57 L58 | L19 L25 L31 L32 | L21 L25 L31 L32 | L22 L34 L35 L36 L37 L42 | L24 L38 L39 L40 | L36 L42 L43 L44 L45 | L39 L46 L47 L48 | L22 L50 L51 A15 | L24 L53 L54 A16 makes body 2 in component "bottom shell"
extrude "Extrude2'" add sketch "bottom_shell" along normal blind 3.6 contours L22 L34 L35 L36 L37 L42 | L24 L38 L39 L40 | L22 L50 L51 A15 | L24 L53 L54 A16 | A12 | A17 bodies 2 in component "bottom shell"
extrude "Extrude3'" add sketch "bottom_shell" along normal blind 2 contours L19 L25 L31 L32 | L21 L25 L31 L32 | L36 L42 L43 L44 L45 | L39 L46 L47 L48 bodies 2 in component "bottom shell"
extrude "Extrude4'" add sketch "bottom_shell" along normal blind 10.6 contours L15 L18 L19 A0 A1 L25 A9 L26 A10 L27 L29 L31 | L15 L19 L20 A2 A3 A8 L25 L27 A11 L28 L32 L33 bodies 2 in component "bottom shell"
extrude "Extrude5'" add sketch "bottom_shell" along normal blind 12.6 contours L21 A5 L22 A6 L23 L25 A9 L26 A10 L27 L29 L31 L34 | A4 L21 L23 A7 L24 A8 L25 L27 A11 L28 L32 L33 bodies 2 in component "bottom shell"
extrude "Extrude6'" add sketch "bottom_shell" along normal blind 1 contours L15 L27 L29 L33 | L23 L27 L29 L33 bodies 2 in component "bottom shell"
extrude "Extrude7'" add sketch "bottom_shell" along normal blind 8 contours L22 A6 L23 L55 L56 | L23 A7 L24 L57 L58 bodies 2 in component "bottom shell"
fillet "Fillet1'" radius 1 12 edges at (17.6, -7.75, -1.8) (25, -7.75, -1.8) (10.3, -7.75, -1.8) (7.8, -7.75, -1.8) (4.3, -7.75, 0.4) (4.3, -0.3, 0.4) (4.3, 61.75, 0.4) (4.3, 54.3, 0.4) (7.8, 61.75, -1.8) (10.3, 61.75, -1.8) (17.6, 61.75, -1.8) (25, 61.75, -1.8) on bodies 2 in component "bottom shell"
fillet "Fillet2" radius 0.5 10 edges at (10.3, -0.3, -0.8) (7.8, -0.3, -0.8) (10.3, 2.2, -2.6) (7.8, 2.2, -2.6) (2.8, -0.3, -3.1) (2.8, 54.3, -3.1) (7.8, 51.8, -2.6) (10.3, 51.8, -2.6) (7.8, 54.3, -0.8) (10.3, 54.3, -0.8) on bodies 2 in component "bottom shell"
sketch "drills" plane through (0.3, 0, 0) normal (-1, 0, 0) x (0, 1, 0) in component "bottom shell"
  circle A0 centre (58, 0.6) radius 1.65 construction
  circle A1 centre (-4, 0.6) radius 1.65 construction
  circle A2 centre (58, -0.6) radius 1.65 construction
  circle A3 centre (-4, -0.6) radius 1.65 construction
  circle A4 centre (-4, -0.6) radius 1.25
  circle A5 centre (58, -0.6) radius 1.25
  dimension "d72" = 2.5
  dimension "d73" = 2.5
  constraint concentric A3 A4
  constraint concentric A2 A5
  measures "d72" diameter of A4
  measures "d73" diameter of A5
extrude "Extrude8'" cut sketch "drills" against normal blind 4 bodies 2 in component "bottom shell"
fillet "Fillet4" radius 0.5 4 edges at (0.3, 56.8346, 0.148) (0.3, -5.1654, 0.148) (4.3, -5.1654, 1.052) (4.3, 56.8346, 1.052) on bodies 2 in component "bottom shell"
ref_plane "WorkPlane1" through (0, 0, 9) normal (0, 0, 1) x (1, 0, 0) in component "top_shell"
sketch "Sketch1" plane through (0, 0, 9) normal (0, 0, 1) x (1, 0, 0) in component "top_shell"
  line L0 (26.8, -10.25) -> (3.3, -10.25)
  arc A0 (26.8, -10.25) -> (29.8, -7.25) centre (26.8, -7.25) ccw
  line L1 (29.8, 61.25) -> (29.8, -7.25)
  line L2 (27.3, 61.25) -> (27.3, -7.25)
  arc A1 (26.8, -7.75) -> (27.3, -7.25) centre (26.8, -7.25) ccw
  line L3 (26.8, -7.75) -> (3.3, -7.75)
  arc A2 (0.3, -7.25) -> (3.3, -10.25) centre (3.3, -7.25) ccw
  line L4 (0.3, 61.25) -> (0.3, -7.25)
  line L5 (2.8, 61.25) -> (2.8, -7.25)
  arc A3 (2.8, -7.25) -> (3.3, -7.75) centre (3.3, -7.25) ccw
  arc A4 (3.3, 64.25) -> (0.3, 61.25) centre (3.3, 61.25) ccw
  line L6 (3.3, 64.25) -> (26.8, 64.25)
  arc A5 (29.8, 61.25) -> (26.8, 64.25) centre (26.8, 61.25) ccw
  arc A6 (27.3, 61.25) -> (26.8, 61.75) centre (26.8, 61.25) ccw
  line L7 (3.3, 61.75) -> (26.8, 61.75)
  arc A7 (3.3, 61.75) -> (2.8, 61.25) centre (3.3, 61.25) ccw
  circle A8 centre (21.3, 58.025) radius 1.75 construction
  circle A9 centre (21.3, -4.025) radius 1.75 construction
  line L8 (2.8, -0.3) -> (0.3, -0.3) construction
  line L9 (27.3, 0.2) -> (29.8, 0.2) construction
  line L10 (27.3, 53.8) -> (29.8, 53.8) construction
  line L11 (2.8, 54.3) -> (0.3, 54.3) construction
  line L12 (8.38, 0.3962) -> (8.38, 6.7463) construction
  line L13 (8.38, 6.7463) -> (8.38, 8.175) construction
  line L14 (8.38, 8.175) -> (8.38, 9.6038) construction
  line L15 (8.38, 9.6038) -> (23.62, 9.6038) construction
  line L16 (14.73, 0.3962) -> (8.38, 0.3962) construction
  line L17 (17.27, 0.3962) -> (14.73, 0.3962) construction
  line L18 (23.62, 0.3962) -> (17.27, 0.3962) construction
  line L19 (23.62, 6.7463) -> (23.62, 0.3962) construction
  line L20 (23.62, 8.175) -> (23.62, 6.7463) construction
  line L21 (23.62, 9.6038) -> (23.62, 8.175) construction
  line L22 (8.08, 0.0962) -> (23.92, 0.0962)
  line L23 (23.92, 0.0962) -> (23.92, 9.9038)
  line L24 (23.92, 9.9038) -> (8.08, 9.9038)
  line L25 (8.08, 9.9038) -> (8.08, 0.0962)
  line L26 (1.3, 61.25) -> (1.3, -7.25)
  arc A10 (1.3, -7.25) -> (3.3, -9.25) centre (3.3, -7.25) ccw
  line L27 (26.8, -9.25) -> (3.3, -9.25)
  arc A11 (26.8, -9.25) -> (28.8, -7.25) centre (26.8, -7.25) ccw
  line L28 (28.8, 61.25) -> (28.8, -7.25)
  arc A12 (28.8, 61.25) -> (26.8, 63.25) centre (26.8, 61.25) ccw
  line L29 (3.3, 63.25) -> (26.8, 63.25)
  arc A13 (3.3, 63.25) -> (1.3, 61.25) centre (3.3, 61.25) ccw
  circle A14 centre (21.3, 58.025) radius 1.25
  circle A15 centre (21.3, 58.025) radius 3
  line L30 (0.3, 27) -> (29.8, 27) construction
  line L31 (27.3, 53.5) -> (29.8, 53.5)
  line L32 (0.3, 54) -> (2.8, 54)
  circle A16 centre (21.3, -4.025) radius 1.25
  circle A17 centre (21.3, -4.025) radius 3
  line L33 (27.3, 0.5) -> (29.8, 0.5)
  line L34 (0.3, 0) -> (2.8, 0)
  dimension "d81" = 0.3
  dimension "d82" = 0.3
  dimension "d83" = 0.3
  dimension "d84" = 0.3
  dimension "d85" = -1
  dimension "d86" = 2.5
  dimension "d87" = 6
  dimension "d90" = 0.3
  dimension "d91" = 0.3
  constraint horizontal L22
  constraint vertical L23
  constraint horizontal L24
  constraint vertical L25
  constraint concentric A8 A14
  constraint concentric A8 A15
  constraint midpoint L4 L30.start
  constraint midpoint L1 L30.end
  constraint coincident L2 L31.start
  constraint coincident L1 L31.end
  constraint perpendicular L1 L31
  constraint coincident L4 L32.start
  constraint coincident L5 L32.end
  constraint perpendicular L5 L32
  constraint symmetric A14 L30 A16
  constraint symmetric A15 L30 A17
  constraint symmetric L30 L31.start L33.start
  constraint symmetric L30 L31.end L33.end
  constraint symmetric L30 L32.start L34.start
  constraint symmetric L30 L32.end L34.end
  measures "d81" distance of L15 L24
  measures "d82" distance of L16 L22
  measures "d83" distance of L12 L25
  measures "d84" distance of L19 L23
  measures "d86" diameter of A14
  measures "d87" diameter of A15
  measures "d90" distance of L11 L32
  measures "d91" distance of L10 L31
extrude "Extrude1''" add sketch "Sketch1" along normal blind 2.5 separate body contours L0 A0 L1 A2 L4 L26 A10 L27 A11 L28 L33 L34 | L1 L28 L31 L33 | L4 L26 L32 L34 | L1 L4 A4 L6 A5 L26 L28 A12 L29 A13 L31 L32 | L2 L28 L31 L33 | L2 A1 L3 L5 A3 L26 A10 L27 A11 L28 L33 L34 | L5 L26 L32 L34 | L2 L5 A6 L7 A7 L26 L28 A12 L29 A13 L31 L32 | L2 A1 L3 L5 A3 A6 L7 A7 | A14 | A15 | A16 | A17 makes body 3 in component "top_shell"
extrude "Extrude2''" add sketch "Sketch1" against normal blind 9 contours L1 L28 L31 L33 | L2 L28 L31 L33 | A15 | A17 bodies 3 in component "top_shell"
extrude "Extrude3''" add sketch "Sketch1" against normal blind 2 contours L0 A0 L1 A2 L4 L26 A10 L27 A11 L28 L33 L34 | L1 L4 A4 L6 A5 L26 L28 A12 L29 A13 L31 L32 bodies 3 in component "top_shell"
extrude "Extrude4''" add sketch "Sketch1" against normal blind 6 contours L4 L26 L32 L34 | L5 L26 L32 L34 bodies 3 in component "top_shell"
fillet "Fillet1''" radius 1 4 edges at (27.3, 0.5, 4.5) (2.8, 0, 6) (27.3, 53.5, 4.5) (2.8, 54, 6) on bodies 3 in component "top_shell"
fillet "Fillet2'" radius 0.5 4 edges at (0.3, 54, 5) (29.8, 53.5, 3.5) (29.8, 0.5, 3.5) (0.3, 0, 5) on bodies 3 in component "top_shell"
fillet "Fillet3" radius 1 2 edges at (18.503, -5.1098, 9) (18.503, 56.9402, 9) on bodies 3 in component "top_shell"
fillet "Fillet4'" radius 0.5 4 edges at (28.8, 53.5, 8) (1.3, 54, 8) (1.3, 0, 8) (28.8, 0.5, 8) on bodies 3 in component "top_shell"
fillet "Fillet5" radius 0.3 4 edges at (8.08, 9.9038, 10.25) (8.08, 0.0962, 10.25) (23.92, 0.0962, 10.25) (23.92, 9.9038, 10.25) on bodies 3 in component "top_shell"
fillet "Fillet6" radius 2 8 edges at (15.05, -10.25, 11.5) (28.9213, -9.3713, 11.5) (29.8, 27, 11.5) (28.9213, 63.3713, 11.5) (15.05, 64.25, 11.5) (1.1787, 63.3713, 11.5) (0.3, 27, 11.5) (1.1787, -9.3713, 11.5) on bodies 3 in component "top_shell"
fillet "Fillet5'" radius 2 8 edges at (15.05, -10.25, -6.1) (1.1787, -9.3713, -6.1) (0.3, 27, -6.1) (1.1787, 63.3713, -6.1) (15.05, 64.25, -6.1) (28.9213, 63.3713, -6.1) (29.8, 27, -6.1) (28.9213, -9.3713, -6.1) on bodies 2 in component "bottom shell"
fillet "Fillet6'" radius 0.5 8 edges at (0.3, 54.3, 2.2) (1.8, 54.3, 8) (0.3, -0.3, 2.2) (2.8, -0.3, 6.7) (29.8, 0.2, 2.7) (27.3, 0.2, 3.7) (27.3, 53.8, 3.7) (29.8, 53.8, 2.7) on bodies 2 in component "bottom shell"
fillet "Fillet8" radius 0.5 3 edges at (1.8, -0.3, 8) (28.3, 0.2, 8) (28.3, 53.8, 8) on bodies 2 in component "bottom shell"
fillet "Fillet9" radius 0.5 42 edges at (26.4, 61.75, -3.6) (25.2929, 61.4571, -3.6) (25, 59.3875, -3.6) (21.3, 54.325, -3.6) (17.6, 59.3875, -3.6) (17.3071, 61.4571, -3.6) (13.95, 61.75, -3.6) (10.5929, 61.4571, -3.6) (10.3, 56.525, -3.6) (10.1536, 51.9464, -3.6) (9.05, 51.8, -3.6) (7.9464, 51.9464, -3.6) (7.8, 56.525, -3.6) (7.5071, 61.4571, -3.6) (6.05, 61.75, -3.6) (4.5929, 61.4571, -3.6) (4.3, 58.025, -3.6) (4.0071, 54.5929, -3.6) (2.9464, 54.1536, -3.6) (2.8, 27, -3.6) (2.9464, -0.1536, -3.6) (4.0071, -0.5929, -3.6) (4.3, -4.025, -3.6) (4.5929, -7.4571, -3.6) (6.05, -7.75, -3.6) (7.5071, -7.4571, -3.6) (7.8, -2.525, -3.6) (7.9464, 2.0536, -3.6) (9.05, 2.2, -3.6) (10.1536, 2.0536, -3.6) (10.3, -2.525, -3.6) (10.5929, -7.4571, -3.6) (13.95, -7.75, -3.6) (17.3071, -7.4571, -3.6) (17.6, -5.3875, -3.6) (21.3, -0.325, -3.6) (25, -5.3875, -3.6) (25.2929, -7.4571, -3.6) (26.4, -7.75, -3.6) (27.1536, -7.6036, -3.6) (27.3, 27, -3.6) (27.1536, 61.6036, -3.6) on bodies 2 in component "bottom shell"
component "PCB" placed x (1, 0, 0) y (0, 1, 0) z (0, 0, 1) at (0, 0, 0)
component "bottom shell" placed x (1, 0, 0) y (0, 1, 0) z (0, 0, 1) at (0, 0, 0)
component "top_shell" placed x (1, 0, 0) y (0, 1, 0) z (0, 0, 1) at (0, 0, 0)
equation "wall = 2.5 mm"
equation "below = pcb + 2 mm"
equation "d26 = -below"
equation "tolerance = 0.3 mm"
equation "d28 = tolerance"
equation "d29 = wall + tolerance"
equation "radius_outline = 3 mm"
equation "d31 = radius_outline"
equation "d32 = radius_outline"
equation "d33 = wall"
equation "d34 = wall * 0.6"
equation "d35 = tolerance"
equation "d37 = wall"
equation "d38 = tolerance"
equation "pcb = 1.6 mm"
equation "d41 = tolerance"
equation "d50 = -wall"
equation "d52 = below"
equation "d54 = below - pcb"
equation "overlap = 2 mm"
equation "bottom_height = below + above"
equation "d58 = bottom_height - overlap"
equation "above = 9 mm"
equation "d61 = bottom_height"
equation "d74 = -wall - 1.5 mm"
equation "d80 = above"
equation "d81 = tolerance"
equation "d82 = tolerance"
equation "d83 = tolerance"
equation "d84 = tolerance"
equation "d85 = -0.4 * wall"
equation "d90 = tolerance"
equation "d91 = tolerance"
equation "d92 = wall"
equation "d94 = -above"
equation "d96 = -overlap"
equation "d98 = -above + 3 mm"
named bodies: "PCB"
